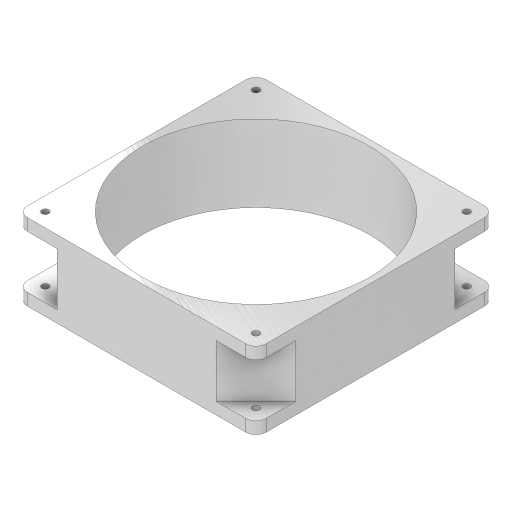
# Autodesk Inventor part: AC-fan-case
Saved by Autodesk Inventor 2024.2 (Build 282272000, 272)
## iProperties
Created: 2023-12-01
Part Number: AC-fan-case
Material: Generic
Document SubType Name: Modeling
Designer: kuzmin
Density: 1 g/cm^3
Appearance: Machined - Aluminum
Author: kuzmin
Autodesk Inventor part; units mm, degrees
ref_plane "YZ Plane" through (0, 0, 0) normal (1, 0, 0) x (0, 1, 0)
ref_plane "XZ Plane" through (0, 0, 0) normal (0, 1, 0) x (-1, 0, 0)
sketch "Sketch1" plane through (0, 0, 0) normal (0, 0, 1) x (1, 0, 0)
  line L0 (-59.6, 59.6) -> (59.6, 59.6)
  line L1 (59.6, 59.6) -> (59.6, -59.6)
  line L2 (59.6, -59.6) -> (-59.6, -59.6)
  line L3 (-59.6, -59.6) -> (-59.6, 59.6)
  point P0 (0, 0)
  point P1 (59.6, 0)
  point P2 (0, 59.6)
  dimension "d0" = 119.2
  constraints: 8 end point, 2 midpoint, 2 parallel, 2 perpendicular, 1 horizontal, 1 horizontal alignment, 1 vertical alignment
  measures "d0" distance of L0.start L0.end
extrude "Extrusion1" add sketch "Sketch1" along normal blind 38.3
fillet "Fillet1" radius 5 4 edges at (-59.6, 59.6, 19.15) (59.6, 59.6, 19.15) (59.6, -59.6, 19.15) (-59.6, -59.6, 19.15)
sketch "Sketch2" plane through (0, 0, 38.3) normal (0, 0, 1) x (1, 0, 0)
  circle A0 centre (52.6, 52.6) radius 1.75
  line L0 (54.6, 59.6) -> (-54.6, 59.6) projected
  line L1 (59.6, -54.6) -> (59.6, 54.6) projected
  point P0 (0, 0)
  dimension "d4" = 7
  dimension "d5" = 7
  dimension "d6" = 3.5
  constraints: 1 centre point
  measures "d4" distance from line of L0 A0.centre
  measures "d5" distance from line of L1 A0.centre
  measures "d6" diameter of A0
extrude "Extrusion2" cut sketch "Sketch2" against normal through all
mirror "Mirror1" about plane through (0, 0, 0) normal (1, 0, 0) of "Extrusion2"
mirror "Mirror2" about plane through (0, 0, 0) normal (0, 1, 0) of "Extrusion2", "Mirror1"
ref_plane "Work Plane1" through (59.6, 59.6, 0) normal (0.7071, -0.7071, 0) x (0, 0, -1)
sketch "Sketch3" plane through (59.6, 59.6, 0) normal (0.7071, -0.7071, 0) x (0, 0, -1)
  line L0 (-32.3, -14.0711) -> (-6, -14.0711)
  line L1 (-6, -14.0711) -> (-6, 12.5661)
  line L2 (-6, 12.5661) -> (-32.3, 12.5661)
  line L3 (-32.3, 12.5661) -> (-32.3, -14.0711)
  line L4 (-38.3, -3.5355) -> (-38.3, -2.0711) projected
  line L5 (0, -2.0711) -> (-38.3, -2.0711) construction
  line L6 (-38.3, -3.5355) -> (-38.3, -80.7516) projected
  line L7 (0, -3.5355) -> (0, -80.7516) projected
  point P0 (0, -84.2871)
  dimension "d9" = 12
  dimension "d10" = 6
  dimension "d11" = 6
  constraints: 8 end point, 2 parallel, 1 horizontal, 1 perpendicular
  measures "d9" distance between parallel lines of L0 L5
  measures "d10" distance between parallel lines of L6 L3
  measures "d11" distance between parallel lines of L7 L1
extrude "Extrusion3" cut sketch "Sketch3" along normal through all both and the other way through all
mirror "Mirror3" about plane through (0, 0, 0) normal (1, 0, 0) of "Extrusion3"
mirror "Mirror4" about plane through (0, 0, 0) normal (0, 1, 0) of "Extrusion3", "Mirror3"
sketch "Sketch4" plane through (0, 0, 38.3) normal (0, 0, 1) x (1, 0, 0)
  circle A0 centre (0, 0) radius 56.75
  dimension "d14" = 113.5
  constraints: 1 centre point, 1 coincident
  measures "d14" diameter of A0
extrude "Extrusion4" cut sketch "Sketch4" against normal through all
body "Solid1"
